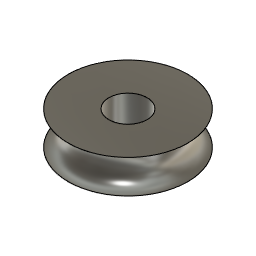
v1 (Autodesk Fusion 360 design; units mm, degrees)
Autodesk Fusion 360 part; units mm, degrees
sketch "草图1" plane through (0, 0, 0) normal (0, 1, 0) x (1, 0, 0)
  line L0 (0, -35) -> (125, -35)
  line L1 (125, 35) -> (0, 35)
  line L2 (0, 35) -> (0, -35)
  arc A0 (125, 35) -> (125, -35) centre (125, 0) ccw
  constraint horizontal L0
  constraint horizontal L1
  constraint vertical L2
revolve "旋转1" add sketch "草图1" angle 360 about axis through (0, 0, -35) along (0, 0, 1)
hole "孔1" at (0, 0, 35) direction (0, 0, -1) diameter 80 depth 100 tip angle 118
sketch "草图2" plane through (0, 0, 0) normal (0, 1, 0) x (1, 0, 0)
